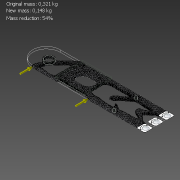
# Autodesk Inventor part: bovenarm - rechts
Saved by Autodesk Inventor 2020 (Build 240168000, 168)
## iProperties
Created: 2020-05-18
Part Number: bovenarm - rechts
Material: Aluminum 6061
Document SubType Name: Modeling
Designer: stefa
Density: 2.7 g/cm^3
Appearance: Aluminum - Polished
Mass: 110.447 g
Surface Area: 239.699 cm^2
Volume: 40.9063 cm^3
Author: stefa
Autodesk Inventor part; units mm, degrees
ref_plane "YZ Plane" through (0, 0, 0) normal (1, 0, 0) x (0, 1, 0)
ref_plane "XZ Plane" through (0, 0, 0) normal (0, 1, 0) x (-1, 0, 0)
ref_plane "XY Plane" through (0, 0, 0) normal (0, 0, 1) x (1, 0, 0)
sketch "Sketch1" plane through (0, 0, 0) normal (0, 1, 0) x (-1, 0, 0)
  line L0 (0, 0) -> (230, 0)
  line L1 (230, 0) -> (230, -50)
  line L2 (230, -50) -> (0, -50)
  line L3 (0, -50) -> (0, 0)
  circle A0 centre (200, -25) radius 7
  line L4 (138.262, -25) -> (128.262, -25) construction
  line L5 (138.262, -13.9) -> (128.262, -13.9)
  line L6 (128.262, -36.1) -> (138.262, -36.1)
  arc A1 (138.262, -36.1) -> (138.262, -13.9) centre (138.262, -25) ccw
  arc A2 (128.262, -13.9) -> (128.262, -36.1) centre (128.262, -25) ccw
  line L7 (153.762, -40.5) -> (143.762, -40.5) construction
  line L8 (153.762, -38.95) -> (143.762, -38.95)
  line L9 (143.762, -42.05) -> (153.762, -42.05)
  arc A3 (153.762, -42.05) -> (153.762, -38.95) centre (153.762, -40.5) ccw
  arc A4 (143.762, -38.95) -> (143.762, -42.05) centre (143.762, -40.5) ccw
  line L10 (112.762, -42.05) -> (122.762, -42.05)
  arc A5 (122.762, -42.05) -> (122.762, -38.95) centre (122.762, -40.5) ccw
  line L11 (122.762, -40.5) -> (112.762, -40.5) construction
  line L12 (122.762, -38.95) -> (112.762, -38.95)
  arc A6 (112.762, -38.95) -> (112.762, -42.05) centre (112.762, -40.5) ccw
  line L13 (143.762, -11.05) -> (153.762, -11.05)
  arc A7 (153.762, -11.05) -> (153.762, -7.95) centre (153.762, -9.5) ccw
  line L14 (153.762, -9.5) -> (143.762, -9.5) construction
  line L15 (153.762, -7.95) -> (143.762, -7.95)
  arc A8 (143.762, -7.95) -> (143.762, -11.05) centre (143.762, -9.5) ccw
  line L16 (112.762, -11.05) -> (122.762, -11.05)
  arc A9 (122.762, -11.05) -> (122.762, -7.95) centre (122.762, -9.5) ccw
  line L17 (122.762, -9.5) -> (112.762, -9.5) construction
  line L18 (122.762, -7.95) -> (112.762, -7.95)
  arc A10 (112.762, -7.95) -> (112.762, -11.05) centre (112.762, -9.5) ccw
  circle A11 centre (160, -45) radius 2
  circle A12 centre (160, -5) radius 2
  circle A13 centre (60, -45) radius 2
  circle A14 centre (60, -5) radius 2
  circle A15 centre (4, -25) radius 2
  circle A16 centre (4, -5) radius 2
  circle A17 centre (4, -45) radius 2
  point P0 (133.262, -25)
  point P1 (148.762, -40.5)
  point P2 (117.762, -40.5)
  point P3 (148.762, -9.5)
  point P4 (117.762, -9.5)
  point P5 (0, -25)
  dimension "d0" = 230
  dimension "d1" = 50
  dimension "d16" = 14
  dimension "d18" = 25
  dimension "d24" = 22.2
  dimension "d25" = 3.1
  dimension "d26" = 10
  dimension "d27" = 10
  dimension "d28" = 66.738
  dimension "d29" = 25
  dimension "d30" = 30
  dimension "d31" = 15.5
  dimension "d32" = 15.5
  dimension "d35" = 31
  dimension "d38" = 31
  dimension "d42" = 4
  dimension "d43" = 70
  dimension "d44" = 5
  dimension "d47" = 40
  dimension "d50" = 100
  dimension "d53" = 4
  dimension "d56" = 4
  dimension "d58" = 20
  dimension "d59" = 20
  constraints: 48 end point, 20 point on circle, 18 centre point, 8 tangent, 5 parallel, 4 horizontal, 3 midpoint, 2 equal radius, 2 vertical, 2 vertical alignment, 1 horizontal alignment, 1 perpendicular, 42 other
  measures "d0" distance of L1.end L2.end
  measures "d1" distance of L0.end L1.end
  measures "d16" diameter of A0
  measures "d18" distance from line of L0 A0.centre
  measures "d24" diameter of A2
  measures "d25" diameter of A4
  measures "d26" distance of L9.start L9.end
  measures "d27" distance of L6.start L6.end
  measures "d28" distance of A0.centre point (133.262, -25)
  measures "d29" distance from line of L0 point (133.262, -25)
  measures "d30" distance from line of L1 A0.centre
  measures "d31" horizontal distance of point (133.262, -25) point (148.762, -40.5)
  measures "d32" horizontal distance of point (148.762, -40.5) point (133.262, -25)
  measures "d35" distance of L9.start L10.start
  measures "d38" distance of L9.start L13.start
  measures "d42" diameter of A11
  measures "d43" distance from line of L1 A11.centre
  measures "d44" distance from line of A11.centre L2
  measures "d47" distance of A11.centre A12.centre
  measures "d50" distance of A11.centre A13.centre
  measures "d53" diameter of A15
  measures "d56" distance from line of L3 A15.centre
  measures "d58" distance of A16.centre A15.centre
  measures "d59" distance of A17.centre A15.centre
extrude "Extrusion1" add sketch "Sketch1" along normal blind 4
fillet "Fillet1" radius 25 2 edges at (-230, 2, 0) (-230, 2, -50)
equation "\"d18\" = 0.5 * d1"
equation "\"d59\" = d58"
body "Solid1"
